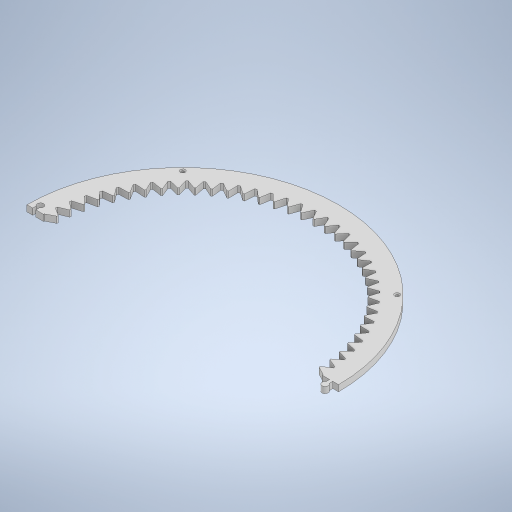
# Autodesk Inventor part: NewBearingGear
Saved by Autodesk Inventor 2023 (Build 270158000, 158)
## iProperties
Created: 2023-03-07
Part Number: NewBearingGear
Material: Generic
Document SubType Name: Modeling
Designer: caleb
Density: 1 g/cm^3
Appearance: Default
Author: caleb
Autodesk Inventor part; units mm, degrees
ref_plane "YZ Plane" through (0, 0, 0) normal (1, 0, 0) x (0, 1, 0)
ref_plane "XZ Plane" through (0, 0, 0) normal (0, 1, 0) x (-1, 0, 0)
ref_plane "XY Plane" through (0, 0, 0) normal (0, 0, 1) x (1, 0, 0)
sketch "Sketch1" plane through (0, 0, 0) normal (0, 1, 0) x (-1, 0, 0)
  circle A0 centre (0, 0) radius 125
  circle A1 centre (0, 0) radius 111.75
  line L0 (0.1489, -111.7499) -> (0.1489, -104.2499)
  line L1 (0.6489, -105.1159) -> (4.4284, -111.6622)
  line L2 (-0.3511, -105.1159) -> (-4.1371, -111.6734)
  line L3 (0.1489, -104.2499) -> (7.7208, -104.2499) construction
  arc A2 (-4.1371, -111.6734) -> (4.4284, -111.6622) centre (0, 0) ccw
  line L4 (0.6489, -105.1159) -> (-0.3511, -105.1159)
  line L5 (125, 0) -> (111.75, 0)
  line L6 (119.125, -5) -> (118.375, 0)
  arc A3 (117.875, -2.8349) -> (120.375, -2.8349) centre (119.125, -5) ccw
  line L7 (121.625, 0) -> (121.625, -5)
  line L8 (116.625, -5) -> (116.625, 0)
  line L9 (119.125, -5) -> (121.625, -5)
  line L10 (120.375, -2.8349) -> (120.375, 0)
  line L11 (117.875, -2.8349) -> (117.875, 0)
  line L12 (120.375, 0) -> (117.875, 0)
  arc A4 (-117.875, 2.8349) -> (-120.375, 2.8349) centre (-119.125, 5) ccw
  line L13 (-120.375, 2.8349) -> (-120.375, 0)
  line L14 (-117.875, 2.8349) -> (-117.875, 0)
  line L15 (-120.375, 0) -> (-117.875, 0)
  line L16 (10.0688, -104.6346) -> (14.4199, -110.8157)
  line L17 (9.0728, -104.7242) -> (5.8899, -111.5947)
  line L18 (10.0688, -104.6346) -> (9.0728, -104.7242)
  line L19 (19.4076, -103.3108) -> (24.2953, -109.077)
  line L20 (18.4237, -103.4894) -> (15.8694, -110.6175)
  line L21 (19.4076, -103.3108) -> (18.4237, -103.4894)
  line L22 (28.5902, -101.1552) -> (33.975, -106.4601)
  line L23 (27.6262, -101.4213) -> (25.7212, -108.7496)
  line L24 (28.5902, -101.1552) -> (27.6262, -101.4213)
  line L25 (37.5426, -98.1852) -> (43.3813, -102.9861)
  line L26 (36.6063, -98.5366) -> (35.3659, -106.0062)
  line L27 (37.5426, -98.1852) -> (36.6063, -98.5366)
  line L28 (46.1927, -94.4246) -> (52.4382, -98.6828)
  line L29 (45.2917, -94.8585) -> (44.7259, -102.4093)
  line L30 (46.1927, -94.4246) -> (45.2917, -94.8585)
  line L31 (54.4709, -89.9038) -> (61.073, -93.585)
  line L32 (53.6124, -90.4167) -> (53.7257, -97.9878)
  line L33 (54.4709, -89.9038) -> (53.6124, -90.4167)
  line L34 (62.3105, -84.6592) -> (69.216, -87.7337)
  line L35 (61.5015, -85.247) -> (62.293, -92.7774)
  line L36 (62.3105, -84.6592) -> (61.5015, -85.247)
  line L37 (69.6485, -78.7329) -> (76.8018, -81.176)
  line L38 (68.8954, -79.3908) -> (70.3587, -86.82)
  line L39 (69.6485, -78.7329) -> (68.8954, -79.3908)
  line L40 (76.4257, -72.1727) -> (83.7692, -73.9648)
  line L41 (75.7346, -72.8955) -> (77.858, -80.1636)
  line L42 (76.4257, -72.1727) -> (75.7346, -72.8955)
  line L43 (82.5875, -65.0314) -> (90.0621, -66.158)
  line L44 (81.964, -65.8132) -> (84.7303, -72.8617)
  line L45 (82.5875, -65.0314) -> (81.964, -65.8132)
  line L46 (88.0844, -57.3665) -> (95.6299, -57.8186)
  line L47 (87.5335, -58.2011) -> (90.9205, -64.9732)
  line L48 (88.0844, -57.3665) -> (87.5335, -58.2011)
  line L49 (92.8721, -49.2398) -> (100.4277, -49.0136)
  line L50 (92.3982, -50.1204) -> (96.3787, -56.5616)
  line L51 (92.8721, -49.2398) -> (92.3982, -50.1204)
  line L52 (96.912, -40.7165) -> (104.417, -39.814)
  line L53 (96.519, -41.6361) -> (101.0608, -47.6946)
  line L54 (96.912, -40.7165) -> (96.519, -41.6361)
  line L55 (100.1717, -31.8655) -> (107.5655, -30.2939)
  line L56 (99.8627, -32.8166) -> (104.9293, -38.4436)
  line L57 (100.1717, -31.8655) -> (99.8627, -32.8166)
  line L58 (102.6248, -22.7579) -> (109.848, -20.5298)
  line L59 (102.4023, -23.7328) -> (107.9529, -28.883)
  line L60 (102.6248, -22.7579) -> (102.4023, -23.7328)
  line L61 (104.2517, -13.4671) -> (111.2461, -10.6005)
  line L62 (104.1175, -14.458) -> (110.1074, -19.0899)
  line L63 (104.2517, -13.4671) -> (104.1175, -14.458)
  line L64 (105.0392, -4.0678) -> (111.7485, -0.5858)
  line L65 (104.9943, -5.0668) -> (111.3753, -9.1431)
  line L66 (105.0392, -4.0678) -> (104.9943, -5.0668)
  line L67 (104.981, 5.3642) -> (111.3511, 9.4336)
  line L68 (105.0258, 4.3652) -> (111.7466, 0.8773)
  line L69 (104.981, 5.3642) -> (105.0258, 4.3652)
  line L70 (104.0775, 14.753) -> (110.0572, 19.3771)
  line L71 (104.2117, 13.7621) -> (111.2181, 10.8906)
  line L72 (104.0775, 14.753) -> (104.2117, 13.7621)
  line L73 (102.3361, 24.0231) -> (107.8772, 29.1645)
  line L74 (102.5586, 23.0482) -> (109.7941, 20.8163)
  line L75 (102.3361, 24.0231) -> (102.5586, 23.0482)
  line L76 (99.7707, 33.0997) -> (104.8286, 38.7172)
  line L77 (100.0797, 32.1487) -> (107.4861, 30.5744)
  line L78 (99.7707, 33.0997) -> (100.0797, 32.1487)
  line L79 (96.402, 41.9098) -> (100.9361, 47.9581)
  line L80 (96.795, 40.9903) -> (104.3128, 40.0863)
  line L81 (96.402, 41.9098) -> (96.795, 40.9903)
  line L82 (92.2571, 50.3825) -> (96.2308, 56.8128)
  line L83 (92.731, 49.5019) -> (100.2995, 49.2754)
  line L84 (92.2571, 50.3825) -> (92.731, 49.5019)
  line L85 (87.3695, 58.4496) -> (90.7507, 65.2102)
  line L86 (87.9204, 57.615) -> (95.4787, 58.0678)
  line L87 (87.3695, 58.4496) -> (87.9204, 57.615)
  line L88 (81.7784, 66.046) -> (84.54, 73.0825)
  line L89 (82.4019, 65.2642) -> (89.8892, 66.3927)
  line L90 (81.7784, 66.046) -> (82.4019, 65.2642)
  line L91 (75.5288, 73.1107) -> (77.6486, 80.3664)
  line L92 (76.2199, 72.3879) -> (83.5759, 74.183)
  line L93 (75.5288, 73.1107) -> (76.2199, 72.3879)
  line L94 (68.6712, 79.5867) -> (70.132, 87.0032)
  line L95 (69.4243, 78.9288) -> (76.5898, 81.3761)
  line L96 (68.6712, 79.5867) -> (69.4243, 78.9288)
  line L97 (61.2607, 85.422) -> (62.0508, 92.9396)
  line L98 (62.0697, 84.8342) -> (68.987, 87.914)
  line L99 (61.2607, 85.422) -> (62.0697, 84.8342)
  line L100 (53.3569, 90.5694) -> (53.4699, 98.1276)
  line L101 (54.2153, 90.0565) -> (60.8287, 93.744)
  line L102 (53.3569, 90.5694) -> (54.2153, 90.0565)
  line L103 (45.0235, 94.9877) -> (44.4586, 102.5256)
  line L104 (45.9245, 94.5538) -> (52.1807, 98.8192)
  line L105 (45.0235, 94.9877) -> (45.9245, 94.5538)
  line L106 (36.3276, 98.6412) -> (35.0893, 106.0981)
  line L107 (37.2638, 98.2898) -> (43.1125, 103.0989)
  line L108 (36.3276, 98.6412) -> (37.2638, 98.2898)
  line L109 (27.3392, 101.5005) -> (25.4375, 108.8163)
  line L110 (28.3032, 101.2344) -> (33.6972, 106.5484)
  line L111 (27.3392, 101.5005) -> (28.3032, 101.2344)
  line L112 (18.1307, 103.5425) -> (15.5809, 110.6585)
  line L113 (19.1147, 103.364) -> (24.0107, 109.14)
  line L114 (18.1307, 103.5425) -> (19.1147, 103.364)
  line L115 (8.7763, 104.7509) -> (5.5988, 111.6097)
  line L116 (9.7722, 104.6613) -> (14.1308, 110.853)
  line L117 (8.7763, 104.7509) -> (9.7722, 104.6613)
  line L118 (-0.6489, 105.1159) -> (-4.4284, 111.6622)
  line L119 (0.3511, 105.1159) -> (4.1371, 111.6734)
  line L120 (-0.6489, 105.1159) -> (0.3511, 105.1159)
  line L121 (-10.0688, 104.6346) -> (-14.4199, 110.8157)
  line L122 (-9.0728, 104.7242) -> (-5.8899, 111.5947)
  line L123 (-10.0688, 104.6346) -> (-9.0728, 104.7242)
  line L124 (-19.4076, 103.3108) -> (-24.2953, 109.077)
  line L125 (-18.4237, 103.4894) -> (-15.8694, 110.6175)
  line L126 (-19.4076, 103.3108) -> (-18.4237, 103.4894)
  line L127 (-28.5902, 101.1552) -> (-33.975, 106.4601)
  line L128 (-27.6262, 101.4213) -> (-25.7212, 108.7496)
  line L129 (-28.5902, 101.1552) -> (-27.6262, 101.4213)
  line L130 (-37.5426, 98.1852) -> (-43.3813, 102.9861)
  line L131 (-36.6063, 98.5366) -> (-35.3659, 106.0062)
  line L132 (-37.5426, 98.1852) -> (-36.6063, 98.5366)
  line L133 (-46.1927, 94.4246) -> (-52.4382, 98.6828)
  line L134 (-45.2917, 94.8585) -> (-44.7259, 102.4093)
  line L135 (-46.1927, 94.4246) -> (-45.2917, 94.8585)
  line L136 (-54.4709, 89.9038) -> (-61.073, 93.585)
  line L137 (-53.6124, 90.4167) -> (-53.7257, 97.9878)
  line L138 (-54.4709, 89.9038) -> (-53.6124, 90.4167)
  line L139 (-62.3105, 84.6592) -> (-69.216, 87.7337)
  line L140 (-61.5015, 85.247) -> (-62.293, 92.7774)
  line L141 (-62.3105, 84.6592) -> (-61.5015, 85.247)
  line L142 (-69.6485, 78.7329) -> (-76.8018, 81.176)
  line L143 (-68.8954, 79.3908) -> (-70.3587, 86.82)
  line L144 (-69.6485, 78.7329) -> (-68.8954, 79.3908)
  line L145 (-76.4257, 72.1727) -> (-83.7692, 73.9648)
  line L146 (-75.7346, 72.8955) -> (-77.858, 80.1636)
  line L147 (-76.4257, 72.1727) -> (-75.7346, 72.8955)
  line L148 (-82.5875, 65.0314) -> (-90.0621, 66.158)
  line L149 (-81.964, 65.8132) -> (-84.7303, 72.8617)
  line L150 (-82.5875, 65.0314) -> (-81.964, 65.8132)
  line L151 (-88.0844, 57.3665) -> (-95.6299, 57.8186)
  line L152 (-87.5335, 58.2011) -> (-90.9205, 64.9732)
  line L153 (-88.0844, 57.3665) -> (-87.5335, 58.2011)
  line L154 (-92.8721, 49.2398) -> (-100.4277, 49.0136)
  line L155 (-92.3982, 50.1204) -> (-96.3787, 56.5616)
  line L156 (-92.8721, 49.2398) -> (-92.3982, 50.1204)
  line L157 (-96.912, 40.7165) -> (-104.417, 39.814)
  line L158 (-96.519, 41.6361) -> (-101.0608, 47.6946)
  line L159 (-96.912, 40.7165) -> (-96.519, 41.6361)
  line L160 (-100.1717, 31.8655) -> (-107.5655, 30.2939)
  line L161 (-99.8627, 32.8166) -> (-104.9293, 38.4436)
  line L162 (-100.1717, 31.8655) -> (-99.8627, 32.8166)
  line L163 (-102.6248, 22.7579) -> (-109.848, 20.5298)
  line L164 (-102.4023, 23.7328) -> (-107.9529, 28.883)
  line L165 (-102.6248, 22.7579) -> (-102.4023, 23.7328)
  line L166 (-104.2517, 13.4671) -> (-111.2461, 10.6005)
  line L167 (-104.1175, 14.458) -> (-110.1074, 19.0899)
  line L168 (-104.2517, 13.4671) -> (-104.1175, 14.458)
  line L169 (-105.0392, 4.0678) -> (-111.7485, 0.5858)
  line L170 (-104.9943, 5.0668) -> (-111.3753, 9.1431)
  line L171 (-105.0392, 4.0678) -> (-104.9943, 5.0668)
  line L172 (-104.981, -5.3642) -> (-111.3511, -9.4336)
  line L173 (-105.0258, -4.3652) -> (-111.7466, -0.8773)
  line L174 (-104.981, -5.3642) -> (-105.0258, -4.3652)
  line L175 (-104.0775, -14.753) -> (-110.0572, -19.3771)
  line L176 (-104.2117, -13.7621) -> (-111.2181, -10.8906)
  line L177 (-104.0775, -14.753) -> (-104.2117, -13.7621)
  line L178 (-102.3361, -24.0231) -> (-107.8772, -29.1645)
  line L179 (-102.5586, -23.0482) -> (-109.7941, -20.8163)
  line L180 (-102.3361, -24.0231) -> (-102.5586, -23.0482)
  line L181 (-99.7707, -33.0997) -> (-104.8286, -38.7172)
  line L182 (-100.0797, -32.1487) -> (-107.4861, -30.5744)
  line L183 (-99.7707, -33.0997) -> (-100.0797, -32.1487)
  line L184 (-96.402, -41.9098) -> (-100.9361, -47.9581)
  line L185 (-96.795, -40.9903) -> (-104.3128, -40.0863)
  line L186 (-96.402, -41.9098) -> (-96.795, -40.9903)
  line L187 (-92.2571, -50.3825) -> (-96.2308, -56.8128)
  line L188 (-92.731, -49.5019) -> (-100.2995, -49.2754)
  line L189 (-92.2571, -50.3825) -> (-92.731, -49.5019)
  line L190 (-87.3695, -58.4496) -> (-90.7507, -65.2102)
  line L191 (-87.9204, -57.615) -> (-95.4787, -58.0678)
  line L192 (-87.3695, -58.4496) -> (-87.9204, -57.615)
  line L193 (-81.7784, -66.046) -> (-84.54, -73.0825)
  line L194 (-82.4019, -65.2642) -> (-89.8892, -66.3927)
  line L195 (-81.7784, -66.046) -> (-82.4019, -65.2642)
  line L196 (-75.5288, -73.1107) -> (-77.6486, -80.3664)
  line L197 (-76.2199, -72.3879) -> (-83.5759, -74.183)
  line L198 (-75.5288, -73.1107) -> (-76.2199, -72.3879)
  line L199 (-68.6712, -79.5867) -> (-70.132, -87.0032)
  line L200 (-69.4243, -78.9288) -> (-76.5898, -81.3761)
  line L201 (-68.6712, -79.5867) -> (-69.4243, -78.9288)
  line L202 (-61.2607, -85.422) -> (-62.0508, -92.9396)
  line L203 (-62.0697, -84.8342) -> (-68.987, -87.914)
  line L204 (-61.2607, -85.422) -> (-62.0697, -84.8342)
  line L205 (-53.3569, -90.5694) -> (-53.4699, -98.1276)
  line L206 (-54.2153, -90.0565) -> (-60.8287, -93.744)
  line L207 (-53.3569, -90.5694) -> (-54.2153, -90.0565)
  line L208 (-45.0235, -94.9877) -> (-44.4586, -102.5256)
  line L209 (-45.9245, -94.5538) -> (-52.1807, -98.8192)
  line L210 (-45.0235, -94.9877) -> (-45.9245, -94.5538)
  line L211 (-36.3276, -98.6412) -> (-35.0893, -106.0981)
  line L212 (-37.2638, -98.2898) -> (-43.1125, -103.0989)
  line L213 (-36.3276, -98.6412) -> (-37.2638, -98.2898)
  line L214 (-27.3392, -101.5005) -> (-25.4375, -108.8163)
  line L215 (-28.3032, -101.2344) -> (-33.6972, -106.5484)
  line L216 (-27.3392, -101.5005) -> (-28.3032, -101.2344)
  line L217 (-18.1307, -103.5425) -> (-15.5809, -110.6585)
  line L218 (-19.1147, -103.364) -> (-24.0107, -109.14)
  line L219 (-18.1307, -103.5425) -> (-19.1147, -103.364)
  line L220 (-8.7763, -104.7509) -> (-5.5988, -111.6097)
  line L221 (-9.7722, -104.6613) -> (-14.1308, -110.853)
  line L222 (-8.7763, -104.7509) -> (-9.7722, -104.6613)
  line L223 (-125, 0) -> (-111.75, 0)
  point P0 (-121.625, 5)
  point P1 (-116.625, 5)
  point P2 (-117.875, 0)
  point P3 (-120.375, 0)
  point P4 (111.7485, -0.5858)
  point P5 (111.3753, -9.1431)
  point P6 (111.2461, -10.6005)
  point P7 (110.1074, -19.0899)
  point P8 (109.848, -20.5298)
  point P9 (107.9529, -28.883)
  point P10 (107.5655, -30.2939)
  point P11 (104.9293, -38.4436)
  point P12 (104.417, -39.814)
  point P13 (101.0608, -47.6946)
  point P14 (100.4277, -49.0136)
  point P15 (96.3787, -56.5616)
  point P16 (95.6299, -57.8186)
  point P17 (90.9205, -64.9732)
  point P18 (90.0621, -66.158)
  point P19 (84.7303, -72.8617)
  point P20 (83.7692, -73.9648)
  point P21 (77.858, -80.1636)
  point P22 (76.8018, -81.176)
  point P23 (70.3587, -86.82)
  point P24 (69.216, -87.7337)
  point P25 (62.293, -92.7774)
  point P26 (61.073, -93.585)
  point P27 (53.7257, -97.9878)
  point P28 (52.4382, -98.6828)
  point P29 (44.7259, -102.4093)
  point P30 (43.3813, -102.9861)
  point P31 (35.3659, -106.0062)
  point P32 (33.975, -106.4601)
  point P33 (25.7212, -108.7496)
  point P34 (24.2953, -109.077)
  point P35 (15.8694, -110.6175)
  point P36 (14.4199, -110.8157)
  point P37 (5.8899, -111.5947)
  point P38 (-5.5988, -111.6097)
  point P39 (-14.1308, -110.853)
  point P40 (-15.5809, -110.6585)
  point P41 (-24.0107, -109.14)
  point P42 (-25.4375, -108.8163)
  point P43 (-33.6972, -106.5484)
  point P44 (-35.0893, -106.0981)
  point P45 (-43.1125, -103.0989)
  point P46 (-44.4586, -102.5256)
  point P47 (-52.1807, -98.8192)
  point P48 (-53.4699, -98.1276)
  point P49 (-60.8287, -93.744)
  point P50 (-62.0508, -92.9396)
  point P51 (-68.987, -87.914)
  point P52 (-70.132, -87.0032)
  point P53 (-76.5898, -81.3761)
  point P54 (-77.6486, -80.3664)
  point P55 (-83.5759, -74.183)
  point P56 (-84.54, -73.0825)
  point P57 (-89.8892, -66.3927)
  point P58 (-90.7507, -65.2102)
  point P59 (-95.4787, -58.0678)
  point P60 (-96.2308, -56.8128)
  point P61 (-100.2995, -49.2754)
  point P62 (-100.9361, -47.9581)
  point P63 (-104.3128, -40.0863)
  point P64 (-104.8286, -38.7172)
  point P65 (-107.4861, -30.5744)
  point P66 (-107.8772, -29.1645)
  point P67 (-109.7941, -20.8163)
  point P68 (-110.0572, -19.3771)
  point P69 (-111.2181, -10.8906)
  point P70 (-111.3511, -9.4336)
  point P71 (-111.7466, -0.8773)
  dimension "d1" = 223.5
  dimension "d0" = 250
  dimension "d2" = 7.5
  dimension "d3" = 30
  dimension "d4" = 120
  dimension "d7" = 1
  dimension "d8" = 1
  dimension "d11" = 360
  dimension "d15" = 360
  constraints: 448 end point, 13 point on circle, 6 point on line, 4 centre point, 4 horizontal, 3 coincident, 3 perpendicular, 2 tangent, 1 collinear, 1 equal length, 1 midpoint, 1 vertical, 521 other
  measures "d0" diameter of A0
  measures "d2" distance of L0.start L0.end
  measures "d3" angle of L0 L1
  measures "d4" angle of L2 L3
  measures "d7" distance of L1.start L0.end
  measures "d8" distance of L2.start L0.end
extrude "Extrusion2" add sketch "Sketch1" along normal blind 5 contours A0 L223 L15 A1 L5 L8 A3 L7 | L7 A3 L10 L5 | L13 A4 L14 L15 | L8 L5 L11 A3 | L173 L174 L172 A1 | A1 L65 L66 L64 | L176 L177 L175 A1 | A1 L62 L63 L61 | L179 L180 L178 A1 | A1 L59 L60 L58 | L182 L183 L181 A1 | A1 L56 L57 L55 | L185 L186 L184 A1 | A1 L53 L54 L52 | L188 L189 L187 A1 | A1 L50 L51 L49 | L191 L192 L190 A1 | A1 L47 L48 L46 | L194 L195 L193 A1 | A1 L44 L45 L43 | L197 L198 L196 A1 | A1 L41 L42 L40 | L200 L201 L199 A1 | A1 L38 L39 L37 | L203 L204 L202 A1 | A1 L35 L36 L34 | L206 L207 L205 A1 | A1 L32 L33 L31 | L209 L210 L208 A1 | A1 L29 L30 L28 | L212 L213 L211 A1 | A1 L26 L27 L25 | L215 L216 L214 A1 | A1 L23 L24 L22 | L218 L219 L217 A1 | A1 L20 L21 L19 | L221 L222 L220 A1 | A1 L17 L18 L16 | L2 L4 L0 A1 | L0 L4 L1 A1
sketch "Sketch2" plane through (0, 5, 0) normal (0, 1, 0) x (1, 0, 0)
  circle A0 centre (0, 0) radius 125 projected
  circle A1 centre (0, 0) radius 111.75 projected
  circle A2 centre (0, 0) radius 118.25
  line L0 (0, 0) -> (88.3883, 88.3883)
  arc A3 (125, 0) -> (-125, 0) centre (0, 0) ccw projected
  line L1 (0, 0) -> (125, 0) construction
  line L2 (88.3883, 88.3883) -> (83.6154, 83.6154)
  circle A4 centre (0, 0) radius 125
  circle A5 centre (0, 0) radius 111.75
  circle A6 centre (0, 0) radius 117.75
  point P0 (86.0019, 86.0019)
  point P1 (-86.0019, 86.0019)
  point P2 (-86.0019, -86.0019)
  point P3 (86.0019, -86.0019)
  dimension "d19" = 236.5
  dimension "d20" = 45
  dimension "d23" = 360
  dimension "d32" = 250
  dimension "d33" = 223.5
  dimension "d34" = 235.5
  constraints: 6 end point, 4 coincident, 3 centre point, 1 equal length, 1 horizontal, 1 midpoint, 1 point on circle, 1 point on line, 8 other
  measures "d20" angle of L1 L0
  measures "d32" diameter of A4
  measures "d33" diameter of A5
  measures "d34" diameter of A6
hole "Hole1" at (-86.0019, 5, -86.0019) at (86.0019, 5, -86.0019) direction (0, -1, 0) diameter 2.4 end through all countersink diameter 4 countersink angle 90
equation "\"d8\" = d7"
body "Solid2"
